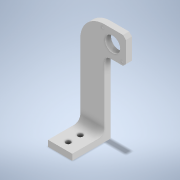
# Autodesk Inventor part: Encoder Mount 1
Saved by Autodesk Inventor 2020 (Build 240168000, 168)
## iProperties
Created: 2020-03-19
Part Number: Encoder Mount 1
Material: Generic
Document SubType Name: Modeling
Designer: DasNick
Density: 1 g/cm^3
Appearance: Default
Author: DasNick
Autodesk Inventor part; units mm, degrees
ref_plane "YZ Plane" through (0, 0, 0) normal (1, 0, 0) x (0, 1, 0)
ref_plane "XZ Plane" through (0, 0, 0) normal (0, 1, 0) x (-1, 0, 0)
sketch "Sketch1" plane through (0, 0, 0) normal (0, 0, 1) x (1, 0, 0)
  point P0 (0, 0)
sketch "Sketch2" plane through (0, 0, 0) normal (0, 0, 1) x (1, 0, 0)
  line L0 (-15.268, 18.9758) -> (-18.9758, 15.268) projected
  spline S0 degree 3 poles (-18.9758, 15.268) (-19.0324, 15.2115) (-19.0821, 15.1506) (-19.1258, 15.0851) (-19.1695, 15.0195) (-19.207, 14.9491) (-19.2371, 14.876) (-19.2671, 14.8029) (-19.2898, 14.727) (-19.3048, 14.6507) (-19.3198, 14.5744) (-19.3273, 14.4976) (-19.3273, 14.4196) knots 0 0 0 0 0.25 0.25 0.25 0.5 0.5 0.5 0.75 0.75 0.75 1 1 1 1 projected
  line L1 (-19.3273, 14.4196) -> (-19.3273, -12.4774) projected
  spline S1 degree 3 poles (-19.3273, -12.4774) (-19.3273, -12.578) (-19.3148, -12.6744) (-19.2919, -12.7664) (-19.2691, -12.8585) (-19.236, -12.9463) (-19.1925, -13.0299) (-19.1491, -13.1135) (-19.0953, -13.1928) (-19.034, -13.2635) (-18.9727, -13.3341) (-18.9038, -13.3961) (-18.8342, -13.4471) (-18.7646, -13.498) (-18.6942, -13.5379) (-18.6223, -13.5705) (-18.5504, -13.6031) (-18.4768, -13.6285) (-18.3951, -13.647) (-18.3133, -13.6656) (-18.2234, -13.6773) (-18.1274, -13.6773) knots 0 0 0 0 0.142857 0.142857 0.142857 0.285714 0.285714 0.285714 0.428571 0.428571 0.428571 0.571429 0.571429 0.571429 0.714286 0.714286 0.714286 0.857143 0.857143 0.857143 1 1 1 1 projected
  line L2 (-18.1274, -13.6773) -> (-15.5, -13.6773) projected
  arc A0 (-13.6773, -15.5) -> (-15.5, -13.6773) centre (-15.5, -15.5) ccw projected
  line L3 (-13.6773, -15.5) -> (-13.6773, -18.1274) projected
  spline S2 degree 3 poles (-13.6773, -18.1274) (-13.6773, -18.228) (-13.6648, -18.3244) (-13.6419, -18.4164) (-13.6191, -18.5085) (-13.586, -18.5963) (-13.5425, -18.6799) (-13.4991, -18.7635) (-13.4453, -18.8428) (-13.384, -18.9135) (-13.3227, -18.9841) (-13.2538, -19.0461) (-13.1842, -19.0971) (-13.1146, -19.148) (-13.0442, -19.1879) (-12.9723, -19.2205) (-12.9004, -19.2531) (-12.8268, -19.2785) (-12.7451, -19.297) (-12.6633, -19.3156) (-12.5734, -19.3273) (-12.4774, -19.3273) knots 0 0 0 0 0.142857 0.142857 0.142857 0.285714 0.285714 0.285714 0.428571 0.428571 0.428571 0.571429 0.571429 0.571429 0.714286 0.714286 0.714286 0.857143 0.857143 0.857143 1 1 1 1 projected
  line L4 (-12.4774, -19.3273) -> (14.4196, -19.3273) projected
  spline S3 degree 3 poles (14.4196, -19.3273) (14.4995, -19.3273) (14.5777, -19.3195) (14.655, -19.3039) (14.7322, -19.2884) (14.8085, -19.2652) (14.8815, -19.2348) (14.9544, -19.2044) (15.0241, -19.1667) (15.0887, -19.1234) (15.1533, -19.08) (15.2128, -19.031) (15.268, -18.9758) knots 0 0 0 0 0.25 0.25 0.25 0.5 0.5 0.5 0.75 0.75 0.75 1 1 1 1 projected
  line L5 (15.268, -18.9758) -> (18.9758, -15.268) projected
  spline S4 degree 3 poles (18.9758, -15.268) (19.0324, -15.2115) (19.0821, -15.1506) (19.1258, -15.0851) (19.1695, -15.0195) (19.207, -14.9491) (19.2371, -14.876) (19.2671, -14.8029) (19.2898, -14.727) (19.3048, -14.6507) (19.3198, -14.5744) (19.3273, -14.4976) (19.3273, -14.4196) knots 0 0 0 0 0.25 0.25 0.25 0.5 0.5 0.5 0.75 0.75 0.75 1 1 1 1 projected
  line L6 (19.3273, -14.4196) -> (19.3273, 12.4774) projected
  spline S5 degree 3 poles (19.3273, 12.4774) (19.3273, 12.578) (19.3148, 12.6744) (19.2919, 12.7664) (19.2691, 12.8585) (19.236, 12.9463) (19.1925, 13.0299) (19.1491, 13.1135) (19.0953, 13.1928) (19.034, 13.2635) (18.9727, 13.3341) (18.9038, 13.3961) (18.8342, 13.4471) (18.7646, 13.498) (18.6942, 13.5379) (18.6223, 13.5705) (18.5504, 13.6031) (18.4768, 13.6285) (18.3951, 13.647) (18.3133, 13.6656) (18.2234, 13.6773) (18.1274, 13.6773) knots 0 0 0 0 0.142857 0.142857 0.142857 0.285714 0.285714 0.285714 0.428571 0.428571 0.428571 0.571429 0.571429 0.571429 0.714286 0.714286 0.714286 0.857143 0.857143 0.857143 1 1 1 1 projected
  line L7 (18.1274, 13.6773) -> (15.5, 13.6773) projected
  arc A1 (13.6773, 15.5) -> (15.5, 13.6773) centre (15.5, 15.5) ccw projected
  line L8 (13.6773, 15.5) -> (13.6773, 18.1274) projected
  spline S6 degree 3 poles (13.6773, 18.1274) (13.6773, 18.228) (13.6648, 18.3244) (13.6419, 18.4164) (13.6191, 18.5085) (13.586, 18.5963) (13.5425, 18.6799) (13.4991, 18.7635) (13.4453, 18.8428) (13.384, 18.9135) (13.3227, 18.9841) (13.2538, 19.0461) (13.1842, 19.0971) (13.1146, 19.148) (13.0442, 19.1879) (12.9723, 19.2205) (12.9004, 19.2531) (12.8268, 19.2785) (12.7451, 19.297) (12.6633, 19.3156) (12.5734, 19.3273) (12.4774, 19.3273) knots 0 0 0 0 0.142857 0.142857 0.142857 0.285714 0.285714 0.285714 0.428571 0.428571 0.428571 0.571429 0.571429 0.571429 0.714286 0.714286 0.714286 0.857143 0.857143 0.857143 1 1 1 1 projected
  line L9 (12.4774, 19.3273) -> (-14.4196, 19.3273) projected
  spline S7 degree 3 poles (-14.4196, 19.3273) (-14.4995, 19.3273) (-14.5777, 19.3195) (-14.655, 19.3039) (-14.7322, 19.2884) (-14.8085, 19.2652) (-14.8815, 19.2348) (-14.9544, 19.2044) (-15.0241, 19.1667) (-15.0887, 19.1234) (-15.1533, 19.08) (-15.2128, 19.031) (-15.268, 18.9758) knots 0 0 0 0 0.25 0.25 0.25 0.5 0.5 0.5 0.75 0.75 0.75 1 1 1 1 projected
  circle A2 centre (-15.5, 15.5) radius 1.5959 projected
  circle A3 centre (15.5, -15.5) radius 1.5959 projected
  circle A4 centre (0, 0) radius 11.9721 projected
  line L10 (21.029, -14.5324) -> (21.029, 14.5324) projected
  line L11 (2.4757, 21.029) -> (14.5324, 21.029) projected
  line L12 (-21.029, -14.5324) -> (-21.029, 14.5324) projected
  line L13 (21.029, 21.029) -> (-21.029, 21.029)
  line L14 (-21.029, 21.029) -> (-21.029, -139.6999)
  line L15 (-21.029, -139.6999) -> (21.029, -139.6999)
  line L16 (21.029, -139.6999) -> (21.029, 21.029)
  line L17 (863.5471, -139.6999) -> (-50.8529, -139.6999)
  point P0 (0, 0)
  dimension "d0" = 0
  dimension "d1" = 0
  constraints: 10 end point, 2 horizontal, 2 parallel, 1 perpendicular, 1 point on line, 2 other
  measures "d0" distance between parallel lines of L17 L15
  measures "d1" distance between parallel lines of L12 L14
extrude "Extrusion1" add sketch "Sketch2" along normal blind 9.525 contours S7 L9 S6 L8 A1 L7 S5 L6 S4 L5 S3 L4 S2 L3 A0 L2 S1 L1 S0 L0 | L16 L15 L14 L12 L13 L11 L10
sketch "Sketch3" plane through (-21.029, -139.6999, 0) normal (-1, 0, 0) x (0, 0, 1)
  line L0 (0, 0) -> (9.525, 0) projected
  line L1 (9.525, 0) -> (9.525, 160.7288)
  line L2 (0, 0) -> (9.525, 0)
  line L3 (9.525, 0) -> (9.525, 167.2458)
  line L4 (9.525, 167.2458) -> (0, 167.2458)
  line L5 (0, 167.2458) -> (0, 0)
  line L6 (0, 160.7288) -> (9.525, 160.7288)
  line L7 (0, 160.7288) -> (9.525, 160.7288) projected
  point P0 (0, 139.6999)
  dimension "d22" = 0
  constraints: 12 end point, 1 horizontal, 1 parallel, 1 point on line
  measures "d22" distance between parallel lines of L7 L6
ref_plane "Work Plane1" through (-50.8529, -184.6081, -243.0428) normal (-1, 0, 0) x (0, 0, 1)
extrude "Extrusion2" add sketch "Sketch3" along normal up to surface (29.8239 mm away) contours L5 L6 L1 L0
sketch "Sketch4" plane through (0, 0, 9.525) normal (0, 0, 1) x (1, 0, 0)
  line L0 (-50.8529, -139.6999) -> (-50.8529, 21.029) projected
  line L1 (-50.8529, -139.6999) -> (-12.7529, -139.6999)
  line L2 (-12.7529, -139.6999) -> (-12.7529, -130.1749)
  line L3 (-12.7529, -130.1749) -> (-50.8529, -130.1749)
  line L4 (-50.8529, -130.1749) -> (-50.8529, -139.6999)
  point P0 (0, 0)
  point P1 (-50.8529, -101.5999)
  dimension "d10" = 9.525
  dimension "d14" = 38.1
  constraints: 8 end point, 2 parallel, 1 horizontal, 1 perpendicular
  measures "d10" distance of L1.end L2.end
  measures "d14" distance between parallel lines of L2 L0
extrude "Extrusion3" add sketch "Sketch4" along normal blind 50.8
fillet "Fillet1" radius 9.525 1 edges at (-31.8029, -130.1749, 9.525)
sketch "Sketch5" plane through (-50.8529, -130.1749, 60.325) normal (0, 1, 0) x (1, 0, 0)
  circle A0 centre (19.05, 31.75) radius 3.9688
  circle A1 centre (19.05, 12.7) radius 3.9688
  line L0 (38.1, 0) -> (0, 0) projected
  point P0 (50.8529, 60.325)
  dimension "d15" = 7.9375
  dimension "d16" = 7.9375
  dimension "d17" = 12.7
  dimension "d18" = 19.05
  constraints: 2 centre point
  measures "d15" diameter of A0
  measures "d16" diameter of A1
  measures "d17" distance from line of L0 A1.centre
  measures "d18" distance of A0.centre A1.centre
extrude "Extrusion4" cut sketch "Sketch5" against normal blind 50.8
sketch "Sketch6" plane through (0, 0, 0) normal (0, 0, -1) x (-1, 0, 0)
  line L0 (50.8529, -139.6999) -> (-21.029, -139.6999)
  line L1 (-21.029, -139.6999) -> (12.7529, -139.6999)
  line L2 (12.7529, -139.6999) -> (12.7529, -21.0043)
  line L3 (12.7529, -21.0043) -> (-21.029, -21.0043)
  line L4 (-21.029, -21.0043) -> (-21.029, -139.6999)
  line L5 (12.7529, -14.5324) -> (12.7529, 14.5324)
  line L6 (50.8529, -139.6999) -> (50.8529, 21.029) projected
  point P0 (0, 0)
  point P1 (12.7529, -139.6999)
  dimension "d23" = 0
  dimension "d24" = 38.1
  constraints: 12 end point
  measures "d23" distance between parallel lines of L5 L2
  measures "d24" distance between parallel lines of L6 L2
extrude "Extrusion5" cut sketch "Sketch6" against normal blind 50.8
fillet "Fillet2" radius 9.525 1 edges at (-12.7529, -21.0043, 4.7625)
chamfer "Chamfer2" distance 4.572 angle 45 2 edges at (21.029, 21.029, 4.7625) (21.029, -21.0043, 4.7625)
fillet "Fillet3" radius 38.1 1 edges at (-50.8529, 21.029, 4.7625)
body "Solid1"
